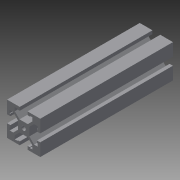
# Autodesk Inventor part: 1_5 80-20 x 6in
Saved by Autodesk Inventor 2014 (Build 180170000, 170)
## iProperties
Created: 2015-02-07
Part Number: 1_5 80-20 x 6in
Material: Generic
Document SubType Name: Modeling
Designer: Spooner
Density: 1 g/cm^3
Appearance: Default
Author: Spooner
Autodesk Inventor part; units mm, degrees
ref_plane "YZ Plane" through (0, 0, 0) normal (1, 0, 0) x (0, 1, 0)
ref_plane "XZ Plane" through (0, 0, 0) normal (0, 1, 0) x (-1, 0, 0)
ref_plane "XY Plane" through (0, 0, 0) normal (0, 0, 1) x (1, 0, 0)
sketch "Sketch1" plane through (0, 0, 0) normal (0, 0, 1) x (1, 0, 0)
  line L0 (6.5405, -6.5405) -> (-6.5405, -6.5405)
  line L1 (-6.5405, -6.5405) -> (-6.5405, 6.5405)
  line L2 (-6.5405, 6.5405) -> (6.5405, 6.5405)
  line L3 (6.5405, 6.5405) -> (6.5405, -6.5405)
  line L4 (6.5405, -6.5405) -> (-6.5405, 6.5405) construction
  line L5 (-6.5405, -6.5405) -> (6.5405, 6.5405) construction
  circle A0 centre (0, 0) radius 2.413
  dimension "d0" = 13.081
  dimension "d1" = 4.826
  constraints: 12 end point, 2 midpoint, 2 parallel, 2 perpendicular, 1 centre point, 1 coincident, 1 horizontal
  measures "d0" distance of L1.end L2.end
  measures "d1" diameter of A0
extrude "Extrusion1" add sketch "Sketch1" along normal blind 152.4
sketch "Sketch2" plane through (0, 0, 152.4) normal (0, 0, 1) x (1, 0, 0)
  circle A0 centre (0, 0) radius 2.413 projected
  line L0 (6.5405, -6.5405) -> (6.5405, 6.5405) projected
  line L1 (19.05, 19.05) -> (19.05, 4.445)
  line L2 (19.05, 4.445) -> (15.24, 4.445)
  line L3 (11.9561, 10.16) -> (6.5405, 4.7444)
  line L4 (15.24, 4.445) -> (15.24, 6.985)
  line L5 (15.24, 6.985) -> (16.002, 6.985)
  line L6 (16.002, 6.985) -> (16.002, 10.16)
  line L7 (16.002, 10.16) -> (11.9561, 10.16)
  line L8 (19.05, 19.05) -> (6.5405, 6.5405) construction
  line L9 (19.05, 19.05) -> (4.445, 19.05)
  line L10 (4.445, 19.05) -> (4.445, 15.24)
  line L11 (10.16, 11.9561) -> (4.7444, 6.5405)
  line L12 (4.445, 15.24) -> (6.985, 15.24)
  line L13 (6.985, 15.24) -> (6.985, 16.002)
  line L14 (6.985, 16.002) -> (10.16, 16.002)
  line L15 (10.16, 16.002) -> (10.16, 11.9561)
  line L16 (4.7444, 6.5405) -> (6.5405, 6.5405)
  line L17 (6.5405, 6.5405) -> (6.5405, 4.7444)
  dimension "d5" = 45
  dimension "d6" = 14.605
  dimension "d7" = 3.81
  dimension "d8" = 3.048
  dimension "d10" = 19.05
  dimension "d13" = 8.89
  dimension "d14" = 1.27
  dimension "d15" = 3.175
  constraints: 34 end point, 7 symmetric about line, 3 perpendicular, 2 parallel, 1 point on line, 1 vertical
  measures "d5" angle of L0 L3
  measures "d6" distance of L1.start L1.end
  measures "d7" distance of L1.end L2.end
  measures "d8" distance between parallel lines of L6 L1
  measures "d10" distance from line of A0.centre L1
  measures "d13" distance from line of L1.start L7
  measures "d14" distance between parallel lines of L8 L3
  measures "d15" distance of L5.end L6.end
extrude "Extrusion2" add sketch "Sketch2" against normal up to surface (152.4 mm away) contours L0 L16 L11 L15 L14 L13 L12 L10 L9 L1 L2 L4 L5 L6 L7 L3
pattern_circular "Circular Pattern1" count 4 over 360 about axis through (0, 0, 0) along (0, 0, 1) of "Extrusion2"
equation "\"d10\" = d9"
equation "\"d9\" = 19.05"
body "Solid1"
